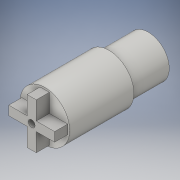
# Autodesk Inventor part: OmniWheelAxleRear
Saved by Autodesk Inventor 2016 (Build 200138000, 138)
## iProperties
Created: 2016-12-01
Part Number: OmniWheelAxleRear
Material: Generic
Document SubType Name: Modeling
Designer: Evan Phil George
Density: 1 g/cm^3
Appearance: Default
Author: Evan Phil George
Autodesk Inventor part; units mm, degrees
ref_plane "YZ Plane" through (0, 0, 0) normal (1, 0, 0) x (0, 1, 0)
ref_plane "XZ Plane" through (0, 0, 0) normal (0, 1, 0) x (-1, 0, 0)
ref_plane "XY Plane" through (0, 0, 0) normal (0, 0, 1) x (1, 0, 0)
sketch "Sketch1" plane through (0, 0, 0) normal (0, 0, 1) x (1, 0, 0)
  circle A0 centre (0, 0) radius 9.5
  dimension "d0" = 19
  constraints: 1 centre point, 1 coincident
  measures "d0" diameter of A0
extrude "Extrusion1" add sketch "Sketch1" against normal blind 24.5
sketch "Sketch2" plane through (0, 0, -24.5) normal (0, 0, -1) x (-1, 0, 0)
  circle A0 centre (0, 0) radius 8
  dimension "d3" = 16
  constraints: 1 centre point, 1 coincident
  measures "d3" diameter of A0
extrude "Extrusion2" add sketch "Sketch2" along normal blind 15
sketch "Sketch3" plane through (0, 0, 0) normal (0, 0, 1) x (1, 0, 0)
  line L0 (0, 0) -> (0, 8.75)
  line L1 (0, 8.75) -> (1.75, 8.75)
  line L2 (1.75, 8.75) -> (1.75, 1.75)
  line L3 (1.75, 1.75) -> (8.75, 1.75)
  line L4 (8.75, 1.75) -> (8.75, -1.75)
  line L5 (8.75, -1.75) -> (1.75, -1.75)
  line L6 (1.75, -1.75) -> (1.75, -8.75)
  line L7 (1.75, -8.75) -> (-1.75, -8.75)
  line L8 (-1.75, -8.75) -> (-1.75, -1.75)
  line L9 (-1.75, -1.75) -> (-8.75, -1.75)
  line L10 (-8.75, -1.75) -> (-8.75, 1.75)
  line L11 (-8.75, 1.75) -> (-1.75, 1.75)
  line L12 (-1.75, 1.75) -> (-1.75, 8.75)
  line L13 (-1.75, 8.75) -> (0, 8.75)
  dimension "d26" = 8.75
  dimension "d27" = 1.75
  dimension "d28" = 7
  dimension "d29" = 7
  dimension "d30" = 3.5
  dimension "d31" = 7
  dimension "d33" = 7
  dimension "d34" = 3.5
  dimension "d35" = 7
  dimension "d36" = 7
  dimension "d37" = 3.5
  dimension "d38" = 7
  dimension "d39" = 7
  constraints: 28 end point, 6 perpendicular, 3 vertical, 2 horizontal, 2 point on line
  measures "d26" distance of L0.start L0.end
  measures "d27" distance of L0.end L1.end
  measures "d28" distance of L1.end L2.end
  measures "d29" distance of L2.end L3.end
  measures "d30" distance of L3.end L4.end
  measures "d31" distance of L4.end L5.end
  measures "d33" distance of L5.end L6.end
  measures "d34" distance of L6.end L7.end
  measures "d35" distance of L7.end L8.end
  measures "d36" distance of L8.end L9.end
  measures "d37" distance of L9.end L10.end
  measures "d38" distance of L10.end L11.end
  measures "d39" distance of L11.end L12.end
extrude "Extrusion3" add sketch "Sketch3" along normal blind 5
sketch "Sketch4" plane through (0, 0, 5) normal (0, 0, 1) x (1, 0, 0)
  circle A0 centre (0, 0) radius 1.3
  dimension "d23" = 2.6
  constraints: 1 centre point, 1 coincident
  measures "d23" diameter of A0
extrude "Extrusion4" cut sketch "Sketch4" against normal blind 42.9375
body "Solid1"
